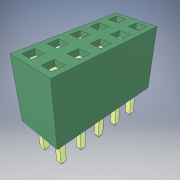
# Autodesk Inventor part: PinHeader-2x5-Female
Saved by Autodesk Inventor 2018 (Build 220112000, 112)
## iProperties
Created: 2021-02-06
Part Number: PinHeader-2x5-Female
Material: Všeobecné
Document SubType Name: Modeling
Designer: Jozko Mrkvicka
Density: 1 g/cm^3
Appearance: Výchozí
Author: Jozko Mrkvicka
Autodesk Inventor part; units mm, degrees
ref_plane "YZ Plane" through (0, 0, 0) normal (1, 0, 0) x (0, 1, 0)
ref_plane "XZ Plane" through (0, 0, 0) normal (0, 1, 0) x (-1, 0, 0)
ref_plane "XY Plane" through (0, 0, 0) normal (0, 0, 1) x (1, 0, 0)
sketch "Náčrt1" plane through (0, 0, 0) normal (0, 1, 0) x (-1, 0, 0)
  line L0 (0, 0) -> (5.08, 0)
  line L1 (5.08, 0) -> (5.08, -12.7)
  line L2 (5.08, -12.7) -> (0, -12.7)
  line L3 (0, -12.7) -> (0, 0)
  dimension "d0" = 5.08
  dimension "d1" = 12.7
  constraints: 8 end point, 2 parallel, 1 horizontal, 1 perpendicular
  measures "d0" distance of L1.end L2.end
  measures "d1" distance of L0.end L1.end
extrude "Vysunutí1" add sketch "Náčrt1" along normal blind 6.985
sketch "Náčrt2" plane through (0, 6.985, 0) normal (0, 1, 0) x (1, 0, 0)
  line L0 (-5.08, 0) -> (0, 0) projected
  line L1 (-5.08, 12.7) -> (-5.08, 0) projected
  line L2 (-4.1275, 0.9525) -> (-3.4925, 0.9525)
  line L3 (-3.4925, 0.9525) -> (-3.4925, 1.5875)
  line L4 (-3.4925, 1.5875) -> (-4.1275, 1.5875)
  line L5 (-4.1275, 1.5875) -> (-4.1275, 0.9525)
  line L6 (-4.1275, 3.4925) -> (-3.4925, 3.4925)
  line L7 (-3.4925, 3.4925) -> (-3.4925, 4.1275)
  line L8 (-3.4925, 4.1275) -> (-4.1275, 4.1275)
  line L9 (-4.1275, 4.1275) -> (-4.1275, 3.4925)
  line L10 (-4.1275, 6.0325) -> (-3.4925, 6.0325)
  line L11 (-3.4925, 6.0325) -> (-3.4925, 6.6675)
  line L12 (-3.4925, 6.6675) -> (-4.1275, 6.6675)
  line L13 (-4.1275, 6.6675) -> (-4.1275, 6.0325)
  line L14 (-4.1275, 8.5725) -> (-3.4925, 8.5725)
  line L15 (-3.4925, 8.5725) -> (-3.4925, 9.2075)
  line L16 (-3.4925, 9.2075) -> (-4.1275, 9.2075)
  line L17 (-4.1275, 9.2075) -> (-4.1275, 8.5725)
  line L18 (-4.1275, 11.1125) -> (-3.4925, 11.1125)
  line L19 (-3.4925, 11.1125) -> (-3.4925, 11.7475)
  line L20 (-3.4925, 11.7475) -> (-4.1275, 11.7475)
  line L21 (-4.1275, 11.7475) -> (-4.1275, 11.1125)
  line L22 (-1.5875, 0.9525) -> (-0.9525, 0.9525)
  line L23 (-0.9525, 0.9525) -> (-0.9525, 1.5875)
  line L24 (-0.9525, 1.5875) -> (-1.5875, 1.5875)
  line L25 (-1.5875, 1.5875) -> (-1.5875, 0.9525)
  line L26 (-1.5875, 3.4925) -> (-0.9525, 3.4925)
  line L27 (-0.9525, 3.4925) -> (-0.9525, 4.1275)
  line L28 (-0.9525, 4.1275) -> (-1.5875, 4.1275)
  line L29 (-1.5875, 4.1275) -> (-1.5875, 3.4925)
  line L30 (-1.5875, 6.0325) -> (-0.9525, 6.0325)
  line L31 (-0.9525, 6.0325) -> (-0.9525, 6.6675)
  line L32 (-0.9525, 6.6675) -> (-1.5875, 6.6675)
  line L33 (-1.5875, 6.6675) -> (-1.5875, 6.0325)
  line L34 (-1.5875, 8.5725) -> (-0.9525, 8.5725)
  line L35 (-0.9525, 8.5725) -> (-0.9525, 9.2075)
  line L36 (-0.9525, 9.2075) -> (-1.5875, 9.2075)
  line L37 (-1.5875, 9.2075) -> (-1.5875, 8.5725)
  line L38 (-1.5875, 11.1125) -> (-0.9525, 11.1125)
  line L39 (-0.9525, 11.1125) -> (-0.9525, 11.7475)
  line L40 (-0.9525, 11.7475) -> (-1.5875, 11.7475)
  line L41 (-1.5875, 11.7475) -> (-1.5875, 11.1125)
  point P0 (-3.81, 1.27)
  dimension "d8" = 2.54
  dimension "d11" = 2.54
  dimension "d17" = 1.27
  dimension "d18" = 1.27
  constraints: 80 end point, 2 horizontal, 2 parallel, 1 perpendicular, 1 vertical, 72 other
  measures "d8" distance of L2.start L6.start
  measures "d11" distance of L2.start L22.start
  measures "d17" distance from line of L0 point (-3.81, 1.27)
  measures "d18" distance from line of L1 point (-3.81, 1.27)
extrude "Vysunutí2" cut sketch "Náčrt2" against normal blind 6.35
sketch "Náčrt3" plane through (0, 6.985, 0) normal (0, 1, 0) x (1, 0, 0)
  line L0 (-0.9525, 9.2075) -> (-0.9525, 8.5725) projected
  line L1 (-0.9525, 8.5725) -> (-1.5875, 8.5725) projected
  line L2 (-1.5875, 8.5725) -> (-1.5875, 9.2075) projected
  line L3 (-1.5875, 9.2075) -> (-0.9525, 9.2075) projected
  line L4 (-0.9525, 4.1275) -> (-0.9525, 3.4925) projected
  line L5 (-0.9525, 3.4925) -> (-1.5875, 3.4925) projected
  line L6 (-1.5875, 3.4925) -> (-1.5875, 4.1275) projected
  line L7 (-1.5875, 4.1275) -> (-0.9525, 4.1275) projected
  line L8 (-3.4925, 11.7475) -> (-3.4925, 11.1125) projected
  line L9 (-3.4925, 11.1125) -> (-4.1275, 11.1125) projected
  line L10 (-4.1275, 11.1125) -> (-4.1275, 11.7475) projected
  line L11 (-4.1275, 11.7475) -> (-3.4925, 11.7475) projected
  line L12 (-3.4925, 6.6675) -> (-3.4925, 6.0325) projected
  line L13 (-3.4925, 6.0325) -> (-4.1275, 6.0325) projected
  line L14 (-4.1275, 6.0325) -> (-4.1275, 6.6675) projected
  line L15 (-4.1275, 6.6675) -> (-3.4925, 6.6675) projected
  line L16 (-3.4925, 1.5875) -> (-3.4925, 0.9525) projected
  line L17 (-3.4925, 0.9525) -> (-4.1275, 0.9525) projected
  line L18 (-4.1275, 0.9525) -> (-4.1275, 1.5875) projected
  line L19 (-4.1275, 1.5875) -> (-3.4925, 1.5875) projected
  line L20 (-3.4925, 4.1275) -> (-3.4925, 3.4925) projected
  line L21 (-3.4925, 3.4925) -> (-4.1275, 3.4925) projected
  line L22 (-4.1275, 3.4925) -> (-4.1275, 4.1275) projected
  line L23 (-4.1275, 4.1275) -> (-3.4925, 4.1275) projected
  line L24 (-3.4925, 9.2075) -> (-3.4925, 8.5725) projected
  line L25 (-3.4925, 8.5725) -> (-4.1275, 8.5725) projected
  line L26 (-4.1275, 8.5725) -> (-4.1275, 9.2075) projected
  line L27 (-4.1275, 9.2075) -> (-3.4925, 9.2075) projected
  line L28 (-0.9525, 1.5875) -> (-0.9525, 0.9525) projected
  line L29 (-0.9525, 0.9525) -> (-1.5875, 0.9525) projected
  line L30 (-1.5875, 0.9525) -> (-1.5875, 1.5875) projected
  line L31 (-1.5875, 1.5875) -> (-0.9525, 1.5875) projected
  line L32 (-0.9525, 6.6675) -> (-0.9525, 6.0325) projected
  line L33 (-0.9525, 6.0325) -> (-1.5875, 6.0325) projected
  line L34 (-1.5875, 6.0325) -> (-1.5875, 6.6675) projected
  line L35 (-1.5875, 6.6675) -> (-0.9525, 6.6675) projected
  line L36 (-0.9525, 11.7475) -> (-0.9525, 11.1125) projected
  line L37 (-0.9525, 11.1125) -> (-1.5875, 11.1125) projected
  line L38 (-1.5875, 11.1125) -> (-1.5875, 11.7475) projected
  line L39 (-1.5875, 11.7475) -> (-0.9525, 11.7475) projected
  line L40 (-5.08, 0) -> (0, 0) projected
  line L41 (-5.08, 12.7) -> (-5.08, 0) projected
  line L42 (-3.175, 0.635) -> (-4.445, 0.635)
  line L43 (-4.445, 0.635) -> (-4.445, 1.905)
  line L44 (-4.445, 1.905) -> (-3.175, 1.905)
  line L45 (-3.175, 1.905) -> (-3.175, 0.635)
  line L46 (-3.175, 0.635) -> (-4.445, 1.905) construction
  line L47 (-4.445, 0.635) -> (-3.175, 1.905) construction
  line L48 (-3.175, 3.175) -> (-4.445, 3.175)
  line L49 (-4.445, 3.175) -> (-4.445, 4.445)
  line L50 (-4.445, 4.445) -> (-3.175, 4.445)
  line L51 (-3.175, 4.445) -> (-3.175, 3.175)
  line L52 (-3.175, 5.715) -> (-4.445, 5.715)
  line L53 (-4.445, 5.715) -> (-4.445, 6.985)
  line L54 (-4.445, 6.985) -> (-3.175, 6.985)
  line L55 (-3.175, 6.985) -> (-3.175, 5.715)
  line L56 (-3.175, 8.255) -> (-4.445, 8.255)
  line L57 (-4.445, 8.255) -> (-4.445, 9.525)
  line L58 (-4.445, 9.525) -> (-3.175, 9.525)
  line L59 (-3.175, 9.525) -> (-3.175, 8.255)
  line L60 (-3.175, 10.795) -> (-4.445, 10.795)
  line L61 (-4.445, 10.795) -> (-4.445, 12.065)
  line L62 (-4.445, 12.065) -> (-3.175, 12.065)
  line L63 (-3.175, 12.065) -> (-3.175, 10.795)
  line L64 (-0.635, 0.635) -> (-1.905, 0.635)
  line L65 (-1.905, 0.635) -> (-1.905, 1.905)
  line L66 (-1.905, 1.905) -> (-0.635, 1.905)
  line L67 (-0.635, 1.905) -> (-0.635, 0.635)
  line L68 (-0.635, 3.175) -> (-1.905, 3.175)
  line L69 (-1.905, 3.175) -> (-1.905, 4.445)
  line L70 (-1.905, 4.445) -> (-0.635, 4.445)
  line L71 (-0.635, 4.445) -> (-0.635, 3.175)
  line L72 (-0.635, 5.715) -> (-1.905, 5.715)
  line L73 (-1.905, 5.715) -> (-1.905, 6.985)
  line L74 (-1.905, 6.985) -> (-0.635, 6.985)
  line L75 (-0.635, 6.985) -> (-0.635, 5.715)
  line L76 (-0.635, 8.255) -> (-1.905, 8.255)
  line L77 (-1.905, 8.255) -> (-1.905, 9.525)
  line L78 (-1.905, 9.525) -> (-0.635, 9.525)
  line L79 (-0.635, 9.525) -> (-0.635, 8.255)
  line L80 (-0.635, 10.795) -> (-1.905, 10.795)
  line L81 (-1.905, 10.795) -> (-1.905, 12.065)
  line L82 (-1.905, 12.065) -> (-0.635, 12.065)
  line L83 (-0.635, 12.065) -> (-0.635, 10.795)
  point P0 (-3.81, 1.27)
  dimension "d21" = 1.27
  dimension "d22" = 1.27
  dimension "d25" = 2.54
  dimension "d28" = 2.54
  constraints: 84 end point, 2 horizontal, 2 midpoint, 2 parallel, 1 perpendicular, 1 vertical, 72 other
  measures "d21" distance of L43.end L44.end
  measures "d22" distance of L42.end L43.end
  measures "d25" distance of L42.start L48.start
  measures "d28" distance of L42.start L64.start
extrude "Vysunutí3" cut sketch "Náčrt3" against normal blind 0.635
sketch "Náčrt4" plane through (0, 0, 0) normal (0, -1, 0) x (1, 0, 0)
  line L0 (-5.08, -12.7) -> (0, -12.7) projected
  line L1 (0, -12.7) -> (0, 0) projected
  line L2 (-0.9525, -11.1125) -> (-0.9525, -11.7475) projected
  line L3 (-0.9525, -11.7475) -> (-1.5875, -11.7475) projected
  line L4 (-1.5875, -11.1125) -> (-0.9525, -11.1125) projected
  line L5 (-1.5875, -11.7475) -> (-1.5875, -11.1125) projected
  line L6 (-1.5875, -11.1125) -> (-1.5875, -11.7475) projected
  line L7 (-0.9525, -11.1125) -> (-1.5875, -11.1125)
  line L8 (-1.5875, -11.1125) -> (-1.5875, -11.7475)
  line L9 (-1.5875, -11.7475) -> (-0.9525, -11.7475)
  line L10 (-0.9525, -11.7475) -> (-0.9525, -11.1125)
  line L11 (-0.9525, -8.5725) -> (-1.5875, -8.5725)
  line L12 (-1.5875, -8.5725) -> (-1.5875, -9.2075)
  line L13 (-1.5875, -9.2075) -> (-0.9525, -9.2075)
  line L14 (-0.9525, -9.2075) -> (-0.9525, -8.5725)
  line L15 (-0.9525, -6.0325) -> (-1.5875, -6.0325)
  line L16 (-1.5875, -6.0325) -> (-1.5875, -6.6675)
  line L17 (-1.5875, -6.6675) -> (-0.9525, -6.6675)
  line L18 (-0.9525, -6.6675) -> (-0.9525, -6.0325)
  line L19 (-0.9525, -3.4925) -> (-1.5875, -3.4925)
  line L20 (-1.5875, -3.4925) -> (-1.5875, -4.1275)
  line L21 (-1.5875, -4.1275) -> (-0.9525, -4.1275)
  line L22 (-0.9525, -4.1275) -> (-0.9525, -3.4925)
  line L23 (-0.9525, -0.9525) -> (-1.5875, -0.9525)
  line L24 (-1.5875, -0.9525) -> (-1.5875, -1.5875)
  line L25 (-1.5875, -1.5875) -> (-0.9525, -1.5875)
  line L26 (-0.9525, -1.5875) -> (-0.9525, -0.9525)
  line L27 (-3.4925, -11.1125) -> (-4.1275, -11.1125)
  line L28 (-4.1275, -11.1125) -> (-4.1275, -11.7475)
  line L29 (-4.1275, -11.7475) -> (-3.4925, -11.7475)
  line L30 (-3.4925, -11.7475) -> (-3.4925, -11.1125)
  line L31 (-3.4925, -8.5725) -> (-4.1275, -8.5725)
  line L32 (-4.1275, -8.5725) -> (-4.1275, -9.2075)
  line L33 (-4.1275, -9.2075) -> (-3.4925, -9.2075)
  line L34 (-3.4925, -9.2075) -> (-3.4925, -8.5725)
  line L35 (-3.4925, -6.0325) -> (-4.1275, -6.0325)
  line L36 (-4.1275, -6.0325) -> (-4.1275, -6.6675)
  line L37 (-4.1275, -6.6675) -> (-3.4925, -6.6675)
  line L38 (-3.4925, -6.6675) -> (-3.4925, -6.0325)
  line L39 (-3.4925, -3.4925) -> (-4.1275, -3.4925)
  line L40 (-4.1275, -3.4925) -> (-4.1275, -4.1275)
  line L41 (-4.1275, -4.1275) -> (-3.4925, -4.1275)
  line L42 (-3.4925, -4.1275) -> (-3.4925, -3.4925)
  line L43 (-3.4925, -0.9525) -> (-4.1275, -0.9525)
  line L44 (-4.1275, -0.9525) -> (-4.1275, -1.5875)
  line L45 (-4.1275, -1.5875) -> (-3.4925, -1.5875)
  line L46 (-3.4925, -1.5875) -> (-3.4925, -0.9525)
  dimension "d35" = 2.54
  dimension "d38" = 2.54
  constraints: 80 end point, 2 horizontal, 2 parallel, 1 perpendicular, 1 vertical, 72 other
  measures "d35" distance of L7.end L11.end
  measures "d38" distance of L7.end L27.end
extrude "Vysunutí4" add sketch "Náčrt4" along normal blind 3.81
chamfer "Zkosení1" distance 0.254 angle 60 4 edges at (-1.27, -3.81, -11.7475) (-1.5875, -3.81, -11.43) (-1.27, -3.81, -11.1125) (-0.9525, -3.81, -11.43) measured on face at (-1.3758, -3.81, -11.3242)
chamfer "Zkosení2" distance 0.254 angle 60 4 edges at (-3.81, -3.81, -11.7475) (-4.1275, -3.81, -11.43) (-3.4925, -3.81, -11.43) (-3.81, -3.81, -11.1125) measured on face at (-3.9158, -3.81, -11.3242)
chamfer "Zkosení3" distance 0.254 angle 60 4 edges at (-4.1275, -3.81, -8.89) (-3.81, -3.81, -9.2075) (-3.4925, -3.81, -8.89) (-3.81, -3.81, -8.5725) measured on face at (-3.9158, -3.81, -8.7842)
chamfer "Zkosení4" distance 0.254 angle 60 4 edges at (-1.5875, -3.81, -8.89) (-1.27, -3.81, -9.2075) (-0.9525, -3.81, -8.89) (-1.27, -3.81, -8.5725) measured on face at (-1.3758, -3.81, -8.7842)
chamfer "Zkosení5" distance 0.254 angle 60 4 edges at (-1.5875, -3.81, -6.35) (-1.27, -3.81, -6.6675) (-0.9525, -3.81, -6.35) (-1.27, -3.81, -6.0325) measured on face at (-1.3758, -3.81, -6.2442)
chamfer "Zkosení6" distance 0.254 angle 60 4 edges at (-4.1275, -3.81, -6.35) (-3.81, -3.81, -6.6675) (-3.4925, -3.81, -6.35) (-3.81, -3.81, -6.0325) measured on face at (-3.9158, -3.81, -6.2442)
chamfer "Zkosení7" distance 0.254 angle 60 4 edges at (-1.5875, -3.81, -3.81) (-1.27, -3.81, -4.1275) (-0.9525, -3.81, -3.81) (-1.27, -3.81, -3.4925) measured on face at (-1.3758, -3.81, -3.7042)
chamfer "Zkosení8" distance 0.254 angle 60 4 edges at (-4.1275, -3.81, -3.81) (-3.81, -3.81, -4.1275) (-3.81, -3.81, -3.4925) (-3.4925, -3.81, -3.81) measured on face at (-3.9158, -3.81, -3.7042)
chamfer "Zkosení9" distance 0.254 angle 60 4 edges at (-1.5875, -3.81, -1.27) (-1.27, -3.81, -1.5875) (-1.27, -3.81, -0.9525) (-0.9525, -3.81, -1.27) measured on face at (-1.3758, -3.81, -1.1642)
chamfer "Zkosení10" distance 0.254 angle 60 4 edges at (-3.81, -3.81, -1.5875) (-4.1275, -3.81, -1.27) (-3.81, -3.81, -0.9525) (-3.4925, -3.81, -1.27) measured on face at (-3.9158, -3.81, -1.1642)
